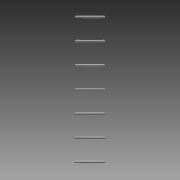
# Autodesk Inventor part: corner cable
Saved by Autodesk Inventor 2015 (Build 190159000, 159)
## iProperties
Created: 2014-05-30
Part Number: corner cable
Material: Steel, Wrought
Document SubType Name: Modeling
Designer: Haden
Density: 7.85 g/cm^3
Appearance: Steel
Author: Haden
Autodesk Inventor part; units mm, degrees
ref_plane "XZ Plane" through (0, 0, 0) normal (0, 1, 0) x (-1, 0, 0)
sketch "Sketch1" plane through (0, 0, 0) normal (0, 0, 1) x (1, 0, 0)
  circle A0 centre (69.85, 0) radius 4.7625
  point P0 (0, 0)
  dimension "d2" = 9.525
  dimension "d3" = 69.85
  constraints: 1 centre point, 1 horizontal alignment
  measures "d2" diameter of A0
  measures "d3" distance of point (0, 0) A0.centre
sketch "Sketch2" plane through (0, 0, 0) normal (1, 0, 0) x (0, 1, 0)
  circle A0 centre (0, 69.85) radius 4.7625
  point P0 (0, 0)
  dimension "d4" = 9.525
  dimension "d5" = 69.85
  constraints: 1 centre point, 1 vertical alignment
  measures "d4" diameter of A0
  measures "d5" distance of point (0, 0) A0.centre
loft "Loft1" add profiles "Sketch2", "Sketch1"
pattern_linear "Rectangular Pattern1" count 7 spacing 101.6 along (0, -1, 0) of "Loft1"
body "Solid1"
